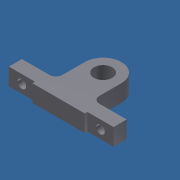
# Autodesk Inventor part: MANCAL DA BETONEIRA(26)
Saved by Autodesk Inventor 2012 SP1 (Build 160190100, 190)
## iProperties
Created: 2012-07-23
Part Number: MANCAL DA BETONEIRA(26)
Material: Carbon Steel
Document SubType Name: Modeling
Designer: bruno.silveira
Mass: 153.953 g
Surface Area: 72.7469 cm^2
Volume: 19.562 cm^3
Density: 7.87 g/cm^3
Author: bruno.silveira
Autodesk Inventor part; units mm, degrees
ref_plane "YZ Plane" through (0, 0, 0) normal (1, 0, 0) x (0, 1, 0)
ref_plane "XZ Plane" through (0, 0, 0) normal (0, 1, 0) x (-1, 0, 0)
ref_plane "XY Plane" through (0, 0, 0) normal (0, 0, 1) x (1, 0, 0)
sketch "Sketch1" plane through (0, 0, 0) normal (0, 0, 1) x (1, 0, 0)
  line L0 (0, 0) -> (80, 0)
  line L1 (80, 0) -> (80, 48)
  line L2 (80, 48) -> (0, 48)
  line L3 (0, 48) -> (0, 0)
  dimension "d0" = 80
  dimension "d1" = 48
  constraints: 8 end point, 2 parallel, 1 horizontal, 1 perpendicular
  measures "d0" distance of L0.start L0.end
  measures "d1" distance of L2.end L0.start
extrude "Extrusion1" add sketch "Sketch1" along normal blind 13
sketch "Sketch2" plane through (0, 0, 13) normal (0, 0, 1) x (1, 0, 0)
  line L0 (80, 0) -> (0, 0) projected
  line L1 (80, 48) -> (80, 0) projected
  point P0 (40, 34)
  dimension "d4" = 34
  dimension "d5" = 40
  measures "d4" distance from line of L0 point (40, 34)
  measures "d5" distance from line of L1 point (40, 34)
hole "Hole1" at (40, 34, 13) direction (0, 0, -1) diameter 14 depth 13 tip angle 118
sketch "Sketch3" plane through (0, 0, 13) normal (0, 0, 1) x (1, 0, 0)
  circle A0 centre (40, 34) radius 7 projected
  line L0 (0, 0) -> (0, 48) projected
  line L1 (80, 0) -> (0, 0) projected
  line L2 (80, 48) -> (80, 0) projected
  line L3 (0, 48) -> (80, 48) projected
  arc A1 (54, 34) -> (26, 34) centre (40, 34) ccw
  line L4 (54, 34) -> (54, 12)
  line L5 (26, 34) -> (26, 12)
  line L6 (0, 12) -> (26, 12)
  line L7 (54, 12) -> (80, 12)
  dimension "d14" = 12
  dimension "d15" = 12
  dimension "d16" = 26
  constraints: 8 end point, 6 perpendicular, 2 point on circle, 2 point on line, 2 tangent, 1 centre point, 1 coincident
  measures "d14" distance between parallel lines of L1 L7
  measures "d15" distance between parallel lines of L1 L6
  measures "d16" distance between parallel lines of L0 L5
extrude "Extrusion2" cut sketch "Sketch3" against normal blind 13 contours L0 L3 A1 L5 L6 | L7 L4 A1 L3 L2
sketch "Sketch4" plane through (0, 0, 13) normal (0, 0, 1) x (1, 0, 0)
  line L0 (0, 0) -> (0, 12) projected
  line L1 (80, 0) -> (0, 0) projected
  line L2 (80, 12) -> (80, 0) projected
  line L3 (0, 2) -> (20, 2)
  line L4 (20, 2) -> (20, 0)
  line L5 (20, 0) -> (0, 0)
  line L6 (0, 0) -> (0, 2)
  line L7 (60, 0) -> (80, 0)
  line L8 (80, 0) -> (80, 2)
  line L9 (80, 2) -> (60, 2)
  line L10 (60, 2) -> (60, 0)
  dimension "d19" = 2
  dimension "d20" = 2
  dimension "d21" = 20
  dimension "d22" = 20
  constraints: 16 end point, 4 parallel, 4 point on line, 2 horizontal, 2 perpendicular
  measures "d19" distance between parallel lines of L7 L9
  measures "d20" distance between parallel lines of L5 L3
  measures "d21" distance of L3.start L3.end
  measures "d22" distance of L8.end L9.end
extrude "Extrusion3" cut sketch "Sketch4" against normal blind 13
sketch "Sketch5" plane through (0, 12, 13) normal (0, 1, 0) x (1, 0, 0)
  line L0 (0, 0) -> (0, 13) projected
  line L1 (26, 0) -> (0, 0) projected
  line L2 (54, 13) -> (80, 13) projected
  line L3 (54, 0) -> (54, 13) projected
  line L4 (80, 0) -> (54, 0) projected
  line L5 (80, 13) -> (80, 0) projected
  point P0 (10, 6.5)
  point P1 (70, 6.5)
  dimension "d25" = 60
  dimension "d26" = 10
  dimension "d27" = 6.5
  measures "d25" distance of point (10, 6.5) point (70, 6.5)
  measures "d26" distance from line of L0 point (10, 6.5)
  measures "d27" distance from line of L1 point (10, 6.5)
hole "Hole2" at (10, 12, 6.5) at (70, 12, 6.5) direction (0, -1, 0) diameter 6.5 depth 10 tip angle 118 counterbore diameter 10 counterbore depth 7
fillet "Fillet1" radius 5 2 edges at (54, 12, 6.5) (26, 12, 6.5)
body "Solid1"
